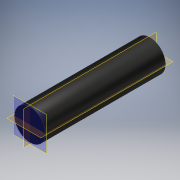
# Autodesk Inventor part: motor-casing
Saved by Autodesk Inventor 2017 (Build 210142000, 142)
## iProperties
Created: 2020-06-17
Part Number: motor-casing
Material: ABS Plastic
Document SubType Name: Modeling
Designer: HAYNIE R&D
Density: 1.06 g/cm^3
Appearance: Smooth - White
Author: HAYNIE R&D
Autodesk Inventor part; units mm, degrees
sketch "Sketch1" plane through (0, 0, 0) normal (0, 1, 0) x (-1, 0, 0)
  circle A0 centre (0, 0) radius 9
  circle A1 centre (0, 0) radius 8
  dimension "d1" = 18
  dimension "d3" = 16
  dimension "d6" = 1
  constraints: 2 centre point, 2 coincident
  measures "d1" diameter of A0
  measures "d3" diameter of A1
  measures "d6" radial gap between concentric circles of A1 A0
extrude "Extrusion1" add sketch "Sketch1" along normal blind 70
sketch "Sketch2" plane through (0, 0, 0) normal (0, -1, 0) x (1, 0, 0)
  circle A0 centre (0, 0) radius 8
  dimension "d7" = 16
  constraints: 1 centre point, 1 coincident
  measures "d7" diameter of A0
extrude "Extrusion2" add sketch "Sketch2" against normal blind 2
body "Solid1"
